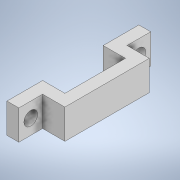
# Autodesk Inventor part: 3d_print_actuator_mount
Saved by Autodesk Inventor 2021 (Build 250183000, 183)
## iProperties
Created: 2021-04-19
Part Number: 3d_print_actuator_mount
Material: Generic
Document SubType Name: Modeling
Designer: Charlie
Density: 1 g/cm^3
Appearance: Default
Author: Charlie
Autodesk Inventor part; units mm, degrees
ref_plane "YZ Plane" through (0, 0, 0) normal (1, 0, 0) x (0, 1, 0)
ref_plane "XZ Plane" through (0, 0, 0) normal (0, 1, 0) x (-1, 0, 0)
ref_plane "XY Plane" through (0, 0, 0) normal (0, 0, 1) x (1, 0, 0)
sketch "Sketch1" plane through (0, 0, 0) normal (0, 1, 0) x (-1, 0, 0)
  line L0 (-3.75, 10.2) -> (3.75, 10.2)
  line L1 (3.75, -10.2) -> (-3.75, -10.2)
  line L2 (-3.75, -10.2) -> (-3.75, 10.2)
  line L3 (-3.75, 10.2) -> (3.75, -10.2) construction
  line L4 (3.75, 10.2) -> (-3.75, -10.2) construction
  line L5 (3.75, 10.2) -> (3.75, 22.2)
  line L6 (-3.75, 0) -> (6.7195, 0) construction
  line L7 (3.75, -10.2) -> (3.75, -22.2)
  line L8 (3.75, 22.2) -> (-0.25, 22.2)
  line L9 (-0.25, 22.2) -> (-0.25, 14.2)
  line L10 (-0.25, 14.2) -> (-7.75, 14.2)
  line L11 (3.75, -22.2) -> (-0.25, -22.2)
  line L12 (-0.25, -22.2) -> (-0.25, -14.2)
  line L13 (-0.25, -14.2) -> (-7.75, -14.2)
  line L14 (-7.75, 14.2) -> (-7.75, -14.2)
  point P0 (0, 0)
  dimension "d0" = 7.5
  dimension "d1" = 20.4
  dimension "d2" = 12
  dimension "d3" = 7.5
  dimension "d5" = 4
  dimension "d6" = 8
  dimension "d7" = 7.5
  constraints: 30 end point, 4 symmetric about line, 3 horizontal, 3 midpoint, 3 perpendicular, 2 vertical, 1 parallel
  measures "d0" distance of L1.start L1.end
  measures "d1" distance of L0.end L1.start
  measures "d2" distance of L0.end L5.end
  measures "d3" distance of L0.start L0.end
  measures "d5" distance of L5.end L8.end
  measures "d6" distance of L8.end L9.end
  measures "d7" distance of L9.end L10.end
extrude "Extrusion1" add sketch "Sketch1" along normal blind 10
sketch "Sketch2" plane through (0.25, 0, 22.2) normal (1, 0, 0) x (0, 0, -1)
  line L0 (22.2, 0) -> (22.2, 12.2527) construction
  line L1 (0, 0) -> (0, 10) construction
  line L2 (8, 0) -> (36.4, 0) construction
  line L3 (0, 10) -> (8, 0) construction
  circle A0 centre (4, 5) radius 2.3
  circle A1 centre (40.4, 5) radius 2.3
  dimension "d10" = 4.6
  constraints: 4 end point, 2 centre point, 1 midpoint, 1 symmetric about line, 1 vertical, 1 other
  measures "d10" diameter of A0
extrude "Extrusion2" cut sketch "Sketch2" against normal through all
body "Solid1"
